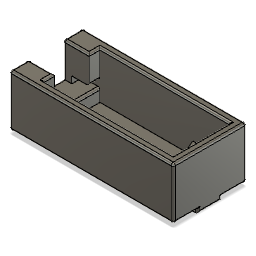
pcb_case (Autodesk Fusion 360 design; units mm, degrees)
Autodesk Fusion 360 part; units mm, degrees
sketch "Sketch1" plane through (0, 0, 0) normal (0, 1, 0) x (1, 0, 0)
  line L0 (17, -6.5) -> (-17, -6.5)
  line L1 (-17, -6.5) -> (-17, 6.5)
  line L2 (-17, 6.5) -> (17, 6.5)
  line L3 (17, 6.5) -> (17, -6.5)
  line L4 (17, -6.5) -> (-17, 6.5) construction
  line L5 (-17, -6.5) -> (17, 6.5) construction
  line L6 (-17, 6.5) -> (-13, 6.5)
  line L7 (-13, 6.5) -> (-13, -6.5)
  line L8 (-13, -6.5) -> (-17, -6.5)
  line L9 (-17, -6.5) -> (-17, 6.5)
  circle A0 centre (14, 0) radius 1.65
  line L10 (19, -8.5) -> (-19, -8.5)
  line L11 (-19, -8.5) -> (-19, 8.5)
  line L12 (-19, 8.5) -> (19, 8.5)
  line L13 (19, 8.5) -> (19, -8.5)
  line L14 (19, -8.5) -> (-19, 8.5) construction
  line L15 (-19, -8.5) -> (19, 8.5) construction
  line L16 (-7.5074, -4.0371) -> (-19.0074, -4.0371)
  line L17 (-19.0074, -4.0371) -> (-19.0074, 3.9629)
  line L18 (-19.0074, 3.9629) -> (-7.5074, 3.9629)
  line L19 (-7.5074, 3.9629) -> (-7.5074, -4.0371)
  line L20 (-7.5074, -4.0371) -> (-19.0074, 3.9629) construction
  line L21 (-19.0074, -4.0371) -> (-7.5074, 3.9629) construction
  point P0 (-13.2574, -0.0371)
  dimension "d1" = 34
  dimension "d2" = 13
  dimension "d3" = 4
  dimension "d4" = 3.3
  dimension "d5" = 38
  dimension "d6" = 17
  dimension "d7" = 11.5
  dimension "d8" = 8
  constraint horizontal L0
  constraint perpendicular L0 L1
  constraint parallel L0 L2
  constraint parallel L1 L3
  constraint coincident L4 origin
  constraint coincident L5 origin
  constraint horizontal L6
  constraint vertical L7
  constraint horizontal L8
  constraint vertical L9
  constraint horizontal L10
  constraint perpendicular L10 L11
  constraint parallel L10 L12
  constraint parallel L11 L13
  constraint coincident L14 origin
  constraint coincident L15 origin
  constraint horizontal L16
  constraint perpendicular L16 L17
  constraint parallel L16 L18
  constraint parallel L17 L19
  constraint coincident L20 P0
  constraint coincident L21 P0
  measures "d1" distance of L1.end L2.end
  measures "d2" distance of L0.end L1.end
  measures "d3" distance of L1.end L6.end
  measures "d4" diameter of A0
  measures "d5" distance of L11.end L12.end
  measures "d6" distance of L10.end L11.end
  measures "d7" distance of L17.end L18.end
  measures "d8" distance of L16.end L17.end
extrude "Extrude1" add sketch "Sketch1" along normal blind 1 contours L0 L1 L2 L3 L6 L8 L9 L10 L11 L12 L13 L16 L18 | L1 L9 L11 L16 L18
extrude "Extrude2" add sketch "Sketch1" along normal blind 1 contours L0 L2 L3 L7 L16 L18 L19 | L0 L1 L7 L8 L9 L16 | L1 L7 L9 L16 L18 | L7 L16 L18 L19 | L1 L2 L6 L7 L9 L18
extrude "Extrude3" add sketch "Sketch1" along normal blind 4 contours L0 L1 L7 L8 L9 L16 | L1 L7 L9 L16 L18 | L1 L2 L6 L7 L9 L18
extrude "Extrude4" add sketch "Sketch1" along normal blind 9 contours L0 L1 L2 L3 L6 L8 L9 L10 L11 L12 L13 L16 L18
extrude "Extrude5" add 1 faces at (-5.6667, 9, -7.8333) along direction (0, 1, 0) blind 3
extrude "Extrude6" add 1 faces at (-17.6667, 1, 1.3704) along direction (0, 1, 0) blind 3
sketch "Sketch3" plane through (0, 1, 0) normal (0, 1, 0) x (-1, 0, 0)
  line L0 (13, 6.5) -> (-17, 6.5)
  line L1 (-17, 6.5) -> (-17, -6.5)
  line L2 (-17, -6.5) -> (13, -6.5)
  line L3 (13, -6.5) -> (13, 6.5)
  circle A0 centre (-14, 0) radius 1.65
  line L4 (-17, -6.5) -> (-8.5, -6.5)
  line L5 (-8.5, -6.5) -> (-8.5, 6.481)
  line L6 (-8.5, 6.481) -> (-17, 6.481)
  line L7 (-17, 6.481) -> (-17, -6.5)
  line L8 (-8.5, -6.5) -> (-11.4437, -0.0095)
  line L9 (-11.4437, -0.0095) -> (-8.5, 6.481)
  dimension "d21" = 8.5
  constraint horizontal L4
  constraint vertical L5
  constraint vertical L7
  constraint coincident L1.end L2.start
  measures "d21" distance of L1.end L4.end
extrude "Extrude7" add sketch "Sketch3" along normal blind 3 contours L1 L2 L4 L6 L7 L8 L9
sketch "Sketch8" plane through (-17, 0, 0) normal (1, 0, 0) x (0, 0, -1)
  line L0 (3.9629, 4) -> (6.5, 4)
  line L1 (6.5, 4) -> (6.5, 12)
  line L2 (6.5, 12) -> (3.9629, 12)
  line L3 (3.9629, 12) -> (3.9629, 4)
  line L4 (3.9629, 12) -> (6.5, 12)
  line L5 (6.5, 12) -> (6.5, 5.57)
  line L6 (6.5, 5.57) -> (3.9629, 5.57)
  line L7 (3.9629, 5.57) -> (3.9629, 12)
  dimension "d34" = 6.43
  constraint horizontal L4
  constraint vertical L5
  constraint horizontal L6
  constraint vertical L7
  constraint coincident L2.end L3.start
  measures "d34" distance of L2.end L6.end
sketch "Sketch9" plane through (-17, 0, 0) normal (1, 0, 0) x (0, 0, -1)
  line L0 (-6.5, 4) -> (-4.0371, 4)
  line L1 (-4.0371, 4) -> (-4.0371, 12)
  line L2 (-4.0371, 12) -> (-6.5, 12)
  line L3 (-6.5, 12) -> (-6.5, 4)
  line L4 (-4.0371, 12) -> (-6.5, 12)
  line L5 (-6.5, 12) -> (-6.5, 5.57)
  line L6 (-6.5, 5.57) -> (-4.0371, 5.57)
  line L7 (-4.0371, 5.57) -> (-4.0371, 12)
  dimension "d35" = 6.43
  constraint horizontal L4
  constraint vertical L5
  constraint horizontal L6
  constraint vertical L7
  constraint coincident L1.end L2.start
  measures "d35" distance of L1.end L6.end
extrude "Extrude9" add sketch "Sketch9" along normal blind 4 contours L1 L2 L3 L4 L5 L6 L7
extrude "Extrude10" add sketch "Sketch8" along normal blind 4 contours L1 L2 L3 L4 L5 L6 L7
sketch "Sketch10" plane through (-19, 0, 0) normal (-1, 0, 0) x (0, 0, 1)
  line L0 (-3.9629, 4) -> (-3.9629, 12)
  line L1 (-3.9629, 12) -> (-8.5, 12)
  line L2 (-8.5, 12) -> (-8.5, 0)
  line L3 (-8.5, 0) -> (8.5, 0)
  line L4 (8.5, 0) -> (8.5, 12)
  line L5 (8.5, 12) -> (4.0371, 12)
  line L6 (4.0371, 12) -> (4.0371, 4)
  line L7 (4.0371, 4) -> (-3.9629, 4)
  line L8 (-2.8, 0.8) -> (2.8, 0.8)
  line L9 (2.8, 0.8) -> (2.8, -0.8)
  line L10 (2.8, -0.8) -> (-2.8, -0.8)
  line L11 (-2.8, -0.8) -> (-2.8, 0.8)
  line L12 (-2.8, 0.8) -> (2.8, -0.8) construction
  line L13 (2.8, 0.8) -> (-2.8, -0.8) construction
  dimension "d40" = 5.6
  dimension "d41" = 1.6
  constraint horizontal L8
  constraint perpendicular L8 L9
  constraint parallel L8 L10
  constraint parallel L9 L11
  constraint coincident L12 origin
  constraint coincident L13 origin
  measures "d40" distance of L9.end L10.end
  measures "d41" distance of L8.end L9.end
extrude "Extrude11" add sketch "Sketch10" against normal blind 38 contours L3 L9 L10 L11
extrude "Extrude12" cut 1 faces at (14.4987, 0, 0.6839) along direction (0, -1, 0) blind 29.5
fillet "Fillet4" radius 0.5 25 edges at (-19, 6, 8.5) (-19, 6, -8.5) (-19, 4, 0.0371) (-19, 8, -3.9629) (-19, 8, 4.0371) (-19, 12, 6.2685) (-19, 12, -6.2315) (-19, 0, 5.65) (-19, 0, -5.65) (0, 12, 8.5) (19, 12, 0) (0, 12, -8.5) (19, 6, 8.5) (19, 6, -8.5) (0, 0, -8.5) (19, 0, -5.65) (19, 0, 5.65) (19, -0.8, 0) (19, -0.4, -2.8) (19, -0.4, 2.8) (12.4617, -0.8, 0.5967) (0, 0, 8.5) (-19, -0.8, 0) (-19, -0.4, 2.8) (-19, -0.4, -2.8)
fillet "Fillet5" radius 0.5 9 edges at (-18.8536, 11.8536, 4.1835) (-15.75, 12, 4.0371) (-18.8536, 11.8536, -4.1094) (-15.75, 12, -3.9629) (-13, 12, 5.2685) (-13, 12, -5.2315) (2, 12, -6.5) (17, 12, 0) (2, 12, 6.5)
fillet "Fillet6" radius 0.5 1 edges at (-13, 4, 0)
fillet "Fillet7" radius 0.5 2 edges at (-13, 5.57, 5.2685) (-13, 5.57, -5.2315)
fillet "Fillet8" radius 0.25 1 edges at (15.5383, 4, 0.5967)
